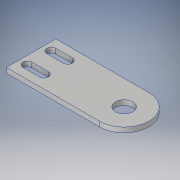
# Autodesk Inventor part: Top Plate
Saved by Autodesk Inventor 2019.4 (Build 234330000, 330)
## iProperties
Created: 2020-01-26
Part Number: Top Plate
Material: Aluminum 6061
Document SubType Name: Modeling
Designer: Mark
Mass: 13.5305 g
Surface Area: 38.3563 cm^2
Volume: 5.01129 cm^3
Density: 2.7 g/cm^3
Appearance: Aluminum - Flat
Author: Mark
Autodesk Inventor part; units mm, degrees
ref_plane "YZ Plane" through (0, 0, 0) normal (1, 0, 0) x (0, 1, 0)
ref_plane "XZ Plane" through (0, 0, 0) normal (0, 1, 0) x (-1, 0, 0)
ref_plane "XY Plane" through (0, 0, 0) normal (0, 0, 1) x (1, 0, 0)
sketch "Sketch1" plane through (0, 0, 0) normal (0, 1, 0) x (-1, 0, 0)
  line L0 (-28.2, 15) -> (28.2, 15)
  line L1 (28.2, 15) -> (28.2, -15)
  line L2 (28.2, -15) -> (-28.2, -15)
  line L3 (-28.2, -15) -> (-28.2, 15)
  line L4 (-28.2, 15) -> (28.2, -15) construction
  line L5 (28.2, 15) -> (-28.2, -15) construction
  arc A0 (-28.2, 15) -> (-28.2, -15) centre (-28.2, 0) ccw
  point P0 (0, 0)
  dimension "d0" = 56.4
  dimension "d1" = 30
  dimension "d2" = 15
  constraints: 12 end point, 2 midpoint, 2 parallel, 2 point on circle, 1 centre point, 1 horizontal, 1 perpendicular
  measures "d0" distance of L1.end L2.end
  measures "d1" distance of L0.end L1.end
  measures "d2" radius of A0
extrude "Extrusion1" add sketch "Sketch1" along normal blind 3
sketch "Sketch2" plane through (0, 3, 0) normal (0, 1, 0) x (1, 0, 0)
  circle A0 centre (28.2, 0) radius 5.25
  arc A1 (28.2, -15) -> (28.2, 15) centre (28.2, 0) ccw projected
  line L0 (-23.2, -7.25) -> (-13.2, -7.25) construction
  line L1 (-23.2, -10) -> (-13.2, -10)
  line L2 (-13.2, -4.5) -> (-23.2, -4.5)
  arc A2 (-23.2, -4.5) -> (-23.2, -10) centre (-23.2, -7.25) ccw
  arc A3 (-13.2, -10) -> (-13.2, -4.5) centre (-13.2, -7.25) ccw
  line L3 (-23.2, -7.25) -> (-13.2, -7.25) construction
  line L4 (-28.2, 15) -> (-28.2, -15) projected
  line L5 (-28.2, -15) -> (28.2, -15) projected
  line L6 (-23.2, 7.25) -> (-13.2, 7.25) construction
  line L7 (-23.2, 4.5) -> (-13.2, 4.5)
  line L8 (-13.2, 10) -> (-23.2, 10)
  arc A4 (-23.2, 10) -> (-23.2, 4.5) centre (-23.2, 7.25) ccw
  arc A5 (-13.2, 4.5) -> (-13.2, 10) centre (-13.2, 7.25) ccw
  line L9 (-23.2, 7.25) -> (-13.2, 7.25) construction
  line L10 (28.2, 15) -> (-28.2, 15) projected
  point P0 (0, 0)
  point P1 (-18.2, -7.25)
  point P2 (-18.2, 7.25)
  dimension "d5" = 10.5
  dimension "d6" = 10
  dimension "d7" = 0
  dimension "d8" = 5.5
  dimension "d9" = 10
  dimension "d10" = 5
  dimension "d11" = 10
  dimension "d12" = 0
  dimension "d13" = 5.5
  dimension "d14" = 5
  dimension "d15" = 10
  constraints: 20 end point, 8 point on circle, 8 tangent, 5 centre point, 4 horizontal, 2 collinear, 2 midpoint, 2 parallel, 1 concentric
  measures "d5" diameter of A0
  measures "d6" distance of L0.start L0.end
  measures "d7" distance between parallel lines of L0 L3
  measures "d8" diameter of A3
  measures "d9" distance from line of L4 point (-18.2, -7.25)
  measures "d10" distance between parallel lines of L5 L1
  measures "d11" distance of L6.start L6.end
  measures "d12" distance between parallel lines of L6 L9
  measures "d13" diameter of A5
  measures "d14" distance between parallel lines of L10 L8
  measures "d15" distance from line of L4 point (-18.2, 7.25)
extrude "Extrusion2" cut sketch "Sketch2" against normal blind 3 contours A0 | A2 L2 A3 L1 | A4 L8 A5 L7
body "Solid1"
